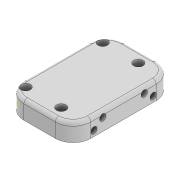
# Autodesk Inventor part: BaseStabilizerAttachment
Saved by Autodesk Inventor 2022 (Build 260153000, 153)
## iProperties
Created: 2022-10-26
Part Number: BaseStabilizerAttachment
Material: Generic
Document SubType Name: Modeling
Designer: MVeszpremi
Density: 1 g/cm^3
Appearance: Default
Author: MVeszpremi
Autodesk Inventor part; units mm, degrees
ref_plane "YZ Plane" through (0, 0, 0) normal (1, 0, 0) x (0, 1, 0)
ref_plane "XZ Plane" through (0, 0, 0) normal (0, 1, 0) x (-1, 0, 0)
ref_plane "XY Plane" through (0, 0, 0) normal (0, 0, 1) x (1, 0, 0)
sketch "Sketch1" plane through (0, 0, 0) normal (0, 1, 0) x (-1, 0, 0)
  line L0 (0, 0) -> (30, 0)
  line L1 (30, 0) -> (30, -65)
  line L2 (30, -65) -> (0, -65)
  line L3 (0, -65) -> (0, 0)
  line L4 (-20, 10) -> (36.5, 10)
  line L5 (36.5, 10) -> (36.5, -75)
  line L6 (36.5, -75) -> (-20, -75)
  line L7 (-20, -75) -> (-20, 10)
  circle A0 centre (30, 0) radius 1.5
  circle A1 centre (30, -65) radius 1.5
  circle A2 centre (0, 0) radius 1.5
  circle A3 centre (0, -65) radius 1.5
  dimension "d0" = 30
  dimension "d1" = 65
  dimension "d2" = 10
  dimension "d3" = 6.5
  dimension "d4" = 10
  dimension "d5" = 20
  dimension "d6" = 3
  dimension "d7" = 3
  dimension "d8" = 3
  dimension "d9" = 3
  constraints: 16 end point, 4 centre point, 4 coincident, 4 parallel, 2 horizontal, 2 perpendicular
  measures "d0" distance of L0.start L0.end
  measures "d1" distance of L0.end L1.end
  measures "d2" distance between parallel lines of L0 L4
  measures "d3" distance between parallel lines of L5 L1
  measures "d4" distance between parallel lines of L6 L2
  measures "d5" distance between parallel lines of L7 L3
  measures "d6" diameter of A0
  measures "d7" diameter of A1
  measures "d8" diameter of A2
  measures "d9" diameter of A3
extrude "Extrusion1" add sketch "Sketch1" along normal blind 15 contours L0 A0 L1 A1 L2 A3 L3 A2 | L4 L5 L6 L7
sketch "Sketch2" plane through (20, 0, 10) normal (1, 0, 0) x (0, 0, -1)
  line L0 (0, 0) -> (0, 15) projected
  line L1 (85, 0) -> (85, 15) projected
  line L2 (42.5, 4.7) -> (42.5, 11.9085)
  circle A0 centre (17.5, 4.7) radius 2.675
  circle A1 centre (67.5, 4.7) radius 2.675
  line L3 (0, 4.7) -> (85, 4.7)
  line L4 (0, 0) -> (85, 0) projected
  line L5 (0, 10.3) -> (85, 10.3)
  circle A2 centre (25, 10.3) radius 2.675
  circle A3 centre (60, 10.3) radius 2.675
  line L6 (0, 15) -> (85, 15) projected
  line L7 (17.5, 7.375) -> (26.8128, 7.375)
  point P0 (10, 0)
  dimension "d12" = 5.35
  dimension "d13" = 5.35
  dimension "d26" = 4.7
  dimension "d27" = 5.35
  dimension "d28" = 5.35
  dimension "d29" = 4.7
  dimension "d31" = 17.5
  dimension "d32" = 17.5
  dimension "d33" = 25
  dimension "d34" = 25
  constraints: 8 end point, 8 point on line, 3 centre point, 2 perpendicular, 1 horizontal, 1 midpoint, 1 vertical, 1 vertical alignment, 2 other
  measures "d13" diameter of A1
  measures "d26" distance between parallel lines of L4 L3
  measures "d27" diameter of A2
  measures "d28" diameter of A3
  measures "d29" distance between parallel lines of L6 L5
  measures "d31" distance from line of A3.centre L2
  measures "d32" distance from line of L2 A2.centre
  measures "d33" distance from line of A1.centre L2
  measures "d34" distance from line of L2 point (17.5, 4.7)
extrude "Extrusion2" cut sketch "Sketch2" against normal blind 43 contours L3 A0 | A0 L3 | A2 L5 | L5 A2 | L3 A1 | A1 L3 | A3 L5 | L5 A3
sketch "Sketch3" plane through (0, 15, 0) normal (0, 1, 0) x (1, 0, 0)
  circle A0 centre (-30, 0) radius 1.5 projected
  circle A1 centre (-30, 0) radius 4
  circle A2 centre (-30, 65) radius 1.5 projected
  circle A3 centre (-30, 65) radius 4
  circle A4 centre (0, 0) radius 1.5 projected
  circle A5 centre (0, 0) radius 4
  circle A6 centre (0, 65) radius 1.5 projected
  circle A7 centre (0, 65) radius 4
  dimension "d18" = 8
  dimension "d19" = 8
  dimension "d20" = 8
  dimension "d21" = 8
  constraints: 4 centre point, 4 coincident
  measures "d18" diameter of A1
  measures "d19" diameter of A3
  measures "d20" diameter of A5
  measures "d21" diameter of A7
extrude "Extrusion3" cut sketch "Sketch3" against normal blind 7.5 contours A0 | A1 | A3 | A5 | A7
fillet "Fillet1" radius 15 4 edges at (-36.5, 7.5, 10) (20, 7.5, 10) (20, 7.5, -75) (-36.5, 7.5, -75)
sketch "Sketch4" plane through (-36.5, 0, -60) normal (-1, 0, 0) x (0, 0, 1)
  point P0 (60, 0)
fillet "Fillet3" radius 3 8 edges at (15.6066, 15, -70.6066) (-8.25, 15, -75) (-32.1066, 15, -70.6066) (-36.5, 15, -32.5) (-32.1066, 15, 5.6066) (-8.25, 15, 10) (15.6066, 15, 5.6066) (20, 15, -32.5)
body "Solid1"
